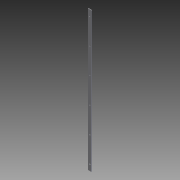
# Autodesk Inventor part: front panels
Saved by Autodesk Inventor 2012 (Build 160160000, 160)
## iProperties
Created: 2012-05-13
Part Number: front panels
Material: Default
Document SubType Name: Modeling
Designer: Puzzles
Density: 1 g/cm^3
Author: Puzzles
Autodesk Inventor part; units mm, degrees
ref_plane "YZ Plane" through (0, 0, 0) normal (1, 0, 0) x (0, 1, 0)
ref_plane "XZ Plane" through (0, 0, 0) normal (0, 1, 0) x (-1, 0, 0)
ref_plane "XY Plane" through (0, 0, 0) normal (0, 0, 1) x (1, 0, 0)
sketch "Sketch1" plane through (0, 0, 0) normal (0, 0, 1) x (1, 0, 0)
  line L0 (-9.525, 381) -> (9.525, 381)
  line L1 (9.525, 381) -> (9.525, -381)
  line L2 (9.525, -381) -> (-9.525, -381)
  line L3 (-9.525, -381) -> (-9.525, 381)
  point P0 (0, 0)
  point P1 (0, 381)
  point P2 (9.525, 0)
  dimension "d0" = 19.05
  dimension "d1" = 762
  constraints: 8 end point, 2 midpoint, 2 parallel, 1 horizontal, 1 horizontal alignment, 1 perpendicular, 1 vertical alignment
  measures "d0" distance of L0.start L0.end
  measures "d1" distance of L2.end L0.start
extrude "Extrusion1" add sketch "Sketch1" along normal blind 3
sketch "Sketch2" plane through (0, 0, 3) normal (0, 0, 1) x (1, 0, 0)
  line L0 (-9.525, 381) -> (9.525, 381) projected
  line L1 (-9.525, -381) -> (-9.525, 381) projected
  line L2 (9.525, -381) -> (-9.525, -381) projected
  point P0 (0, 0)
  point P1 (0, 349.25)
  point P2 (0, 209.55)
  point P3 (0, 69.85)
  point P4 (0, -69.85)
  point P5 (0, -209.55)
  point P6 (0, -349.25)
  dimension "d4" = 12.7
  dimension "d5" = 31.75
  dimension "d6" = 139.7
  dimension "d7" = 139.7
  dimension "d9" = 139.7
  dimension "d10" = 139.7
  dimension "d11" = 139.7
  dimension "d12" = 31.75
  measures "d5" distance from line of L0 point (0, 349.25)
  measures "d6" distance of point (0, 209.55) point (0, 349.25)
  measures "d7" distance of point (0, 69.85) point (0, 209.55)
  measures "d9" distance of point (0, -69.85) point (0, 69.85)
  measures "d10" distance of point (0, -209.55) point (0, -69.85)
  measures "d11" distance of point (0, -349.25) point (0, -209.55)
  measures "d12" distance from line of L2 point (0, -349.25)
hole "Hole1" at (0, 349.25, 3) at (0, 209.55, 3) at (0, 69.85, 3) at (0, -69.85, 3) at (0, -209.55, 3) at (0, -349.25, 3) direction (0, 0, -1) diameter 6.35 end through all
body "Solid1"
